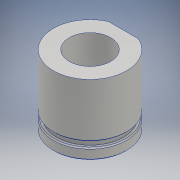
# Autodesk Inventor part: bocal_de_aquecimento
Saved by Autodesk Inventor 2018 (Build 220112000, 112)
## iProperties
Created: 2018-05-10
Part Number: bocal_de_aquecimento
Material: Alumínio 6061
Document SubType Name: Modeling
Designer: Georgines
Density: 2.7 g/cm^3
Appearance: Alumínio - Plano
Mass: 379.718 g
Surface Area: 264.222 cm^2
Volume: 140.636 cm^3
Author: Georgines
Autodesk Inventor part; units mm, degrees
sketch "Esboço2" plane through (0, 0, 0) normal (0, 1, 0) x (-1, 0, 0)
  line L0 (0, 0) -> (-19.2, 0) construction
  line L1 (-34, 1) -> (-34, 9)
  line L2 (-33, 10) -> (-31, 10)
  line L3 (-31, 10) -> (-31, 15)
  line L4 (-31, 15) -> (-33, 15)
  line L5 (-34, 16) -> (-34, 65)
  line L6 (0, 0) -> (0, 69.2361) construction
  line L7 (-34, 65) -> (-19.2, 65)
  line L8 (-19.2, 0) -> (-19.2, 1)
  line L9 (-19.2, 1) -> (-29.5, 1)
  line L10 (-29.5, 1) -> (-29.5, 0)
  line L11 (-29.5, 0) -> (-33, 0)
  line L12 (-19.2, 1) -> (-19.2, 65)
  line L13 (-34, 16) -> (-33, 15)
  line L14 (-34, 9) -> (-33, 10)
  line L15 (-34, 1) -> (-33, 0)
  point P0 (-34, 0)
  point P1 (-34, 10)
  point P2 (-34, 15)
  dimension "d1" = 19.2
  dimension "d6" = 14.8
  dimension "d7" = 10
  dimension "d8" = 3
  dimension "d9" = 5
  dimension "d11" = 50
  dimension "d14" = 1
  dimension "d15" = 10.3
  dimension "d16" = 1
  dimension "d17" = 1
  dimension "d18" = 1
  dimension "d19" = 1
  dimension "d20" = 1
  dimension "d21" = 1
  constraints: 32 end point, 8 point on line, 5 perpendicular, 3 vertical, 1 horizontal, 1 parallel
  measures "d1" distance of L0.start L0.end
  measures "d6" distance of L0.end point (-34, 0)
  measures "d7" distance of point (-34, 0) point (-34, 10)
  measures "d8" distance of point (-34, 10) L2.end
  measures "d9" distance of L2.end L3.end
  measures "d11" distance of point (-34, 15) L5.end
  measures "d14" distance of L0.end L8.end
  measures "d15" distance of L8.end L9.end
  measures "d16" distance of L5.start point (-34, 15)
  measures "d17" distance of L4.end point (-34, 15)
  measures "d18" distance of L1.end point (-34, 10)
  measures "d19" distance of L2.start point (-34, 10)
  measures "d20" distance of L1.start point (-34, 0)
  measures "d21" distance of L11.end point (-34, 0)
revolve "Revolução1" add sketch "Esboço2" angle 360 about axis through (0, 0, 0) along (0, 0, 1)
ref_plane "Plano de trabalho1" through (0, 0, 65) normal (0, 0, 1) x (1, 0, 0)
sketch "Esboço3" plane through (0, 0, 65) normal (0, 0, 1) x (1, 0, 0)
  line L0 (0, 0) -> (0, 19.06) construction
  line L1 (0, 19.06) -> (0, 31.06) construction
  line L2 (0, 31.06) -> (33, 31.06) construction
  line L3 (33, 31.06) -> (33, 44.9163)
  line L4 (33, 44.9163) -> (-33, 44.9163)
  line L5 (-33, 44.9163) -> (-33, 31.06)
  line L6 (-33, 31.06) -> (33, 31.06)
  dimension "d30" = 12
  dimension "d31" = 19.06
  constraints: 14 end point, 3 perpendicular, 3 vertical, 1 collinear
  measures "d30" distance of L0.end L1.end
  measures "d31" distance of L0.start L0.end
extrude "Extrusão1" cut sketch "Esboço3" against normal blind 38
ref_plane "Plano de trabalho2" through (-13.8302, 31.06, 65) normal (0, 1, 0) x (1, 0, 0)
sketch "Esboço5" plane through (-13.8302, 31.06, 65) normal (0, 1, 0) x (1, 0, 0)
  line L0 (0, 0) -> (0, 38) projected
  line L1 (27.6605, 0) -> (0, 0) projected
  line L2 (27.6605, 38) -> (27.6605, 0) projected
  line L3 (5, 5) -> (5, 33)
  line L4 (5, 33) -> (22.6605, 33)
  line L5 (22.6605, 33) -> (22.6605, 5)
  line L6 (22.6605, 5) -> (5, 5)
  line L7 (27.6605, 38) -> (0, 38) projected
  point P0 (13.8302, 65)
  dimension "d33" = 5
  constraints: 8 end point, 1 other
  measures "d33" distance between parallel lines of L1 L6
hole "Furo1" at (8.8302, 31.06, 60) at (8.8302, 31.06, 32) at (-8.8302, 31.06, 32) at (-8.8302, 31.06, 60) direction (0, -1, 0) diameter 3.242 depth 8 tip angle 118 thread size "M4x0.7" class "6H" standard "ISO Metric profile"
ref_plane "Plano de trabalho3" through (0, 0, 1) normal (0, 0, -1) x (-1, 0, 0)
sketch "Esboço7" plane through (0, 0, 1) normal (0, 0, -1) x (-1, 0, 0)
  circle A0 centre (0, 0) radius 19.2 construction
  circle A1 centre (0, 0) radius 29.2679 construction
  circle A2 centre (0, 0) radius 19.2 projected
  line L0 (-19.2, 0) -> (-24.367, 0) construction
  circle A3 centre (-24.367, 0) radius 4.1
  circle A4 centre (12.1835, -21.1024) radius 4.1
  circle A5 centre (12.1835, 21.1024) radius 4.1
  dimension "d42" = 5.167
  dimension "d43" = 8.2
  dimension "d46" = 360
  constraints: 5 centre point, 3 coincident, 2 end point, 1 horizontal, 1 horizontal alignment, 8 other
  measures "d42" distance of L0.start L0.end
  measures "d43" diameter of A3
extrude "Extrusão2" cut sketch "Esboço7" against normal blind 2.2 contours A3 | A4 | A5
ref_plane "Plano de trabalho4" through (-13.8302, 31.06, 65) normal (0, 1, 0) x (1, 0, 0)
ref_plane "Plano de trabalho5" through (0, 34, 27) normal (0, 1, 0) x (-1, 0, 0)
sketch "Esboço10" plane through (0, 34, 27) normal (0, 1, 0) x (-1, 0, 0)
  line L0 (-13.8302, 0) -> (13.8302, 0) projected
  line L1 (0, 0) -> (0, -27) construction
  line L2 (0, -27) -> (0, -24) construction
  dimension "d53" = 3
  constraints: 4 end point, 1 midpoint, 1 point on line, 1 vertical
  measures "d53" distance of L1.end L2.end
hole "Furo2" at (0, 34, 3) direction (0, -1, 0) diameter 3.2 depth 17.2 tip angle 118
equation "\"d17\" = d16"
equation "\"d18\" = d16"
equation "\"d19\" = d18"
equation "\"d20\" = d16"
equation "\"d21\" = d20"
